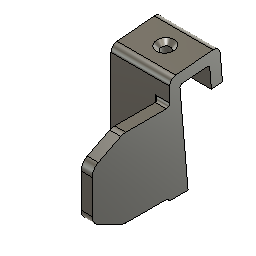
toolholder bracket v3 (Autodesk Fusion 360 design; units mm, degrees)
Autodesk Fusion 360 part; units mm, degrees
note: some values were not read from the file. Set by a fixed rule: which sketch regions a step uses.
sketch "Sketch1" plane through (0, 0, 0) normal (0, 0, 1) x (1, 0, 0)
  line L0 (0, 0) -> (0, 38)
  line L1 (0, 38) -> (26.5, 38)
  line L2 (26.5, 38) -> (26.5, 0)
  line L3 (26.5, 0) -> (0, 0)
  line L4 (21.5, 36.75) -> (26.5, 36.75)
  line L5 (26.5, 36.75) -> (26.5, 1.25)
  line L6 (26.5, 1.25) -> (21.5, 1.25)
  line L7 (21.5, 1.25) -> (21.5, 36.75)
  dimension "d1" = 38
  dimension "d2" = 26.5
  dimension "d9" = 26.5
  dimension "d10" = 21.5
  dimension "d11" = 1.25
  dimension "d12" = 1.25
  constraint coincident L0.start L3.end
  constraint vertical L0
  constraint perpendicular L0 L1
  constraint perpendicular L1 L2
  constraint perpendicular L0 L3
  constraint horizontal L4
  constraint vertical L5
  constraint horizontal L6
  constraint vertical L7
  measures "d1" distance of L0.start L0.end
  measures "d2" distance of L0.end L1.end
  measures "d9" distance of L0 L5
  measures "d10" distance of L0 L7
  measures "d11" distance of L1 L4
  measures "d12" distance of L3 L6
sketch "Sketch2" plane through (0, 0, 0) normal (1, 0, 0) x (0, 0, -1)
  line L0 (0, 0) -> (0, 38)
  line L1 (0, 38) -> (5, 38)
  line L2 (5, 38) -> (8.3246, 0)
  line L3 (5, 38) -> (45, 38) construction
  line L4 (0, 0) -> (8.3246, 0)
  line L5 (5, 38) -> (4.6514, 41.9848)
  line L6 (5, 38) -> (9.981, 38) construction
  line L7 (5.5604, 43.0681) -> (17.0167, 44.0704)
  line L8 (18.1, 43.1614) -> (18.8844, 34.1956)
  line L9 (18.8844, 34.1956) -> (23.8654, 34.6314)
  line L10 (23.8654, 34.6314) -> (22.558, 49.5743)
  line L11 (22.558, 49.5743) -> (0, 47.6008)
  line L12 (0, 47.6008) -> (0, 38)
  arc A0 (18.1, 43.1614) -> (17.0167, 44.0704) centre (17.1038, 43.0742) ccw
  arc A1 (5.5604, 43.0681) -> (4.6514, 41.9848) centre (5.6476, 42.0719) ccw
  point P0 (4.5642, 42.981)
  point P1 (18.0128, 44.1576)
  dimension "d14" = 5
  dimension "d15" = 85
  dimension "d17" = 95
  dimension "d18" = 5
  dimension "d19" = 13.5
  dimension "d20" = 10
  dimension "d21" = 5
  dimension "d22" = 15
  dimension "d36" = 1
  dimension "d37" = 1
  constraint coincident L0.end L1.start
  constraint perpendicular L0 L1
  constraint horizontal L3
  constraint coincident L0.start L4.start
  constraint perpendicular L0 L4
  constraint horizontal L6
  constraint perpendicular L5 L7
  constraint perpendicular L7 L8
  constraint perpendicular L8 L9
  constraint perpendicular L9 L10
  constraint perpendicular L10 L11
  constraint perpendicular L1 L12
  constraint coincident P1 L7
  constraint coincident P1 L8
  constraint tangent L7 A0
  constraint tangent L8 A0
  constraint coincident P0 L7
  constraint coincident P0 L5
  constraint tangent L7 A1
  constraint tangent L5 A1
  measures "d14" distance of L0.end L1.end
  measures "d15" angle of L2 L3
  measures "d17" angle of L5 L6
  measures "d18" distance of L1.end P0
  measures "d19" distance of P0 P1
  measures "d20" distance of P1 L8.end
  measures "d21" distance of L8.end L9.end
  measures "d22" distance of L9.end L10.end
  measures "d36" radius of A0
  measures "d37" radius of A1
extrude "Extrude1" add sketch "Sketch2" along normal up to surface (26.5 mm away)
extrude "Extrude2" add sketch "Sketch1" along normal blind 35 contours L2 L4 L5 L6 L7
sketch "Sketch3" plane through (26.5, 0, 0) normal (1, 0, 0) x (0, 0, -1)
  line L0 (0, 0) -> (8.3246, 0)
  line L1 (8.3246, 0) -> (4.6514, 41.9848)
  line L2 (5.5604, 43.0681) -> (17.0167, 44.0704)
  line L3 (18.1, 43.1614) -> (18.8844, 34.1956)
  line L4 (18.8844, 34.1956) -> (23.8654, 34.6314)
  line L5 (23.8654, 34.6314) -> (22.558, 49.5743)
  line L6 (22.558, 49.5743) -> (0, 47.6008)
  line L7 (0, 47.6008) -> (0, 36.75)
  line L8 (0, 36.75) -> (-35, 36.75)
  line L9 (-35, 36.75) -> (-35, 1.25)
  line L10 (-35, 1.25) -> (0, 1.25)
  line L11 (0, 1.25) -> (0, 0)
  line L12 (-35, 29.75) -> (-21, 36.75)
  line L13 (-35, 19) -> (0, 19) construction
  line L14 (-35, 8.25) -> (-21, 1.25)
  arc A0 (18.1, 43.1614) -> (17.0167, 44.0704) centre (17.1038, 43.0742) ccw
  arc A1 (5.5604, 43.0681) -> (4.6514, 41.9848) centre (5.6476, 42.0719) ccw
  dimension "d27" = 7
  dimension "d28" = 14
  constraint coincident L9 L12.start
  constraint coincident L8 L12.end
  constraint midpoint L9 L13.start
  constraint perpendicular L9 L13
  constraint symmetric L12.start L13 L14.start
  constraint symmetric L12.end L13 L14.end
  measures "d27" distance of L8.end L12.start
  measures "d28" distance of L8.end L12.end
extrude "Extrude3" cut sketch "Sketch3" against normal blind 20 contours L9 L10 L14 | L8 L9 L12
sketch "Sketch4" plane through (0, 47.2392, 4.1329) normal (0, 0.996195, 0.087156) x (1, 0, 0)
  line L0 (26.5, 4.1487) -> (26.5, 26.7929)
  line L1 (26.5, 26.7929) -> (0, 26.7929)
  line L2 (0, 26.7929) -> (0, 4.1487)
  line L3 (0, 4.1487) -> (26.5, 4.1487)
  line L4 (0, 26.7929) -> (26.5, 4.1487)
  line L5 (26.5, 26.7929) -> (0, 4.1487)
  point P0 (13.25, 15.4708)
  constraint coincident L1.end L2.start
  constraint coincident L0.start L3.end
  constraint coincident L0.end L1.start
  constraint coincident L2.end L3.start
  constraint midpoint L4 P0
hole "Hole1" at (13.25, 48.5875, -11.279) direction (0, -0.996195, -0.087156) diameter 4.2 depth 20 tip angle 118 countersink diameter 8 countersink angle 90
fillet "Fillet1" radius 5 4 edges at (24, 36.75, 21) (24, 1.25, 21) (24, 8.25, 35) (24, 29.75, 35)
fillet "Fillet2" radius 3 2 edges at (13.25, 47.6008, 0) (13.25, 49.5743, -22.558)
fillet "Fillet3" radius 1.5 3 edges at (24, 1.25, 0) (21.5, 19, 0) (24, 36.75, 0)
